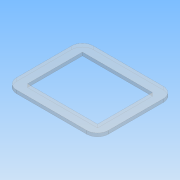
# Autodesk Inventor part: Front_stopper2
Saved by Autodesk Inventor 2016 (Build 200138000, 138)
## iProperties
Created: 2016-04-04
Part Number: Front_stopper2
Material: Polycarbonate, Clear
Document SubType Name: Modeling
Designer: admin
Density: 1.2 g/cm^3
Appearance: Polycarbonate - Clear
Author: admin
Autodesk Inventor part; units mm, degrees
ref_plane "YZ Plane" through (0, 0, 0) normal (1, 0, 0) x (0, 1, 0)
ref_plane "XZ Plane" through (0, 0, 0) normal (0, 1, 0) x (-1, 0, 0)
ref_plane "XY Plane" through (0, 0, 0) normal (0, 0, 1) x (1, 0, 0)
sketch "Sketch1" plane through (0, 0, 0) normal (0, 0, 1) x (1, 0, 0)
  line L0 (-32.5, 25.5) -> (32.5, 25.5)
  line L1 (32.5, 25.5) -> (32.5, -25.5)
  line L2 (32.5, -25.5) -> (-32.5, -25.5)
  line L3 (-32.5, -25.5) -> (-32.5, 25.5)
  line L4 (-32.5, 35.5) -> (32.5, 35.5)
  line L5 (42.5, 25.5) -> (42.5, -25.5)
  line L6 (32.5, -35.5) -> (-32.5, -35.5)
  line L7 (-42.5, -25.5) -> (-42.5, 25.5)
  arc A0 (-32.5, 35.5) -> (-42.5, 25.5) centre (-32.5, 25.5) ccw
  arc A1 (-42.5, -25.5) -> (-32.5, -35.5) centre (-32.5, -25.5) ccw
  arc A2 (32.5, -35.5) -> (42.5, -25.5) centre (32.5, -25.5) ccw
  arc A3 (42.5, 25.5) -> (32.5, 35.5) centre (32.5, 25.5) ccw
  point P0 (0, 0)
  point P1 (0, 25.5)
  point P2 (32.5, 0)
  point P3 (42.5, 0)
  point P4 (0, 35.5)
  dimension "d0" = 65
  dimension "d1" = 51
  dimension "d2" = 10
  dimension "d3" = 10
  dimension "d4" = 10
  constraints: 16 end point, 8 point on circle, 8 tangent, 4 centre point, 4 midpoint, 4 parallel, 3 equal radius, 2 horizontal, 2 horizontal alignment, 2 perpendicular, 2 vertical alignment
  measures "d0" distance of L1.end L2.end
  measures "d1" distance of L0.end L1.end
  measures "d2" radius of A0
  measures "d3" distance between parallel lines of L7 L3
  measures "d4" distance between parallel lines of L4 L0
extrude "Extrusion1" add sketch "Sketch1" along normal blind 3
equation "\"d4\" = d3"
body "Solid1"
